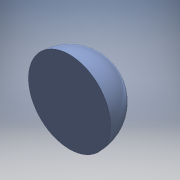
# Autodesk Inventor part: Pied
Saved by Autodesk Inventor 2016 SP1 (Build 200210100, 210)
## iProperties
Created: 2016-01-29
Part Number: Pied
Material: Caoutchouc
Document SubType Name: Modeling
Designer: dimercur
Mass: 0.243473 g
Surface Area: 2.35619 cm^2
Volume: 0.261799 cm^3
Density: 0.93 g/cm^3
Appearance: Caoutchouc - Bleu
Author: dimercur
Autodesk Inventor part; units mm, degrees
ref_plane "YZ Plane" through (0, 0, 0) normal (1, 0, 0) x (0, 1, 0)
ref_plane "XZ Plane" through (0, 0, 0) normal (0, 1, 0) x (-1, 0, 0)
ref_plane "XY Plane" through (0, 0, 0) normal (0, 0, 1) x (1, 0, 0)
sketch "Esquisse1" plane through (0, 0, 0) normal (0, 1, 0) x (-1, 0, 0)
  circle A0 centre (0, 0) radius 5
  dimension "d0" = 10
  constraints: 1 centre point, 1 coincident
  measures "d0" diameter of A0
extrude "Extrusion1" add sketch "Esquisse1" along normal blind 5
fillet "Congé1" radius 5 1 edges at (5, 5, 0)
